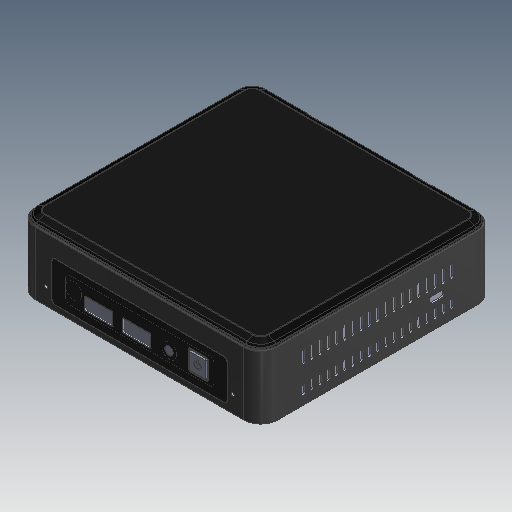
# Autodesk Inventor part: NUC7i5-7BNK-CHASSIS
Saved by Autodesk Inventor 2019.4 (Build 234330000, 330)
## iProperties
Created: 2017-02-08
Part Number: NUC7i5-7BNK-CHASSIS
Material: 一般
Description: STEP AP214
Document SubType Name: Modeling
Designer: y6tada
Density: 1 g/cm^3
Appearance: 既定
Mass: 0.0424115 g
Surface Area: 1.41372 cm^2
Volume: 0.0424115 cm^3
Sending System: SolidWorks 2015
Preprocessor: SwSTEP 2.0
Title: NUC_BN_i5i7_Simplified Chassis.STEP
Revision Number: ANY
Autodesk Inventor part; units mm, degrees
ref_plane "YZ Plane" through (0, 0, 0) normal (1, 0, 0) x (0, 1, 0)
ref_plane "XZ Plane" through (0, 0, 0) normal (0, 1, 0) x (-1, 0, 0)
ref_plane "XY Plane" through (0, 0, 0) normal (0, 0, 1) x (1, 0, 0)
surface "コンポジット1"
sketch "スケッチ1" plane through (-49.5, -3.2, -55.5) normal (0, -1, 0) x (1, 0, 0)
  line L0 (49.5, 98) -> (49.5, 13) construction
  circle A0 centre (49.5, 98) radius 1.5
  circle A1 centre (49.5, 13) radius 1.5
  circle A2 centre (49.5, 98) radius 3
  circle A3 centre (49.5, 13) radius 3
  circle A4 centre (2, 100.9) radius 5.4197 projected
  circle A5 centre (97, 100.9) radius 5.4197 projected
  circle A6 centre (97, 10.1) radius 5.4197 projected
  circle A7 centre (2, 10.1) radius 5.4197 projected
  arc A8 (0, 111) -> (-8, 103) centre (0, 103) ccw projected
  point P0 (49.5, 55.5)
  point P1 (49.5, 55.5)
  dimension "d0" = 85
  dimension "d1" = 3
  dimension "d2" = 6
  constraints: 5 coincident, 4 centre point, 2 end point, 2 equal radius, 1 midpoint, 1 vertical
  measures "d0" distance of L0.start L0.end
  measures "d1" diameter of A0
  measures "d2" diameter of A2
extrude "押し出し1" add sketch "スケッチ1" along normal blind 1 contours A2 | A3
body "Srf1"
